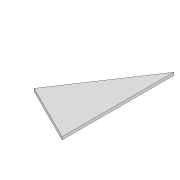
# Autodesk Inventor part: marker
Saved by Autodesk Inventor 2022 (Build 260153000, 153)
## iProperties
Created: 2022-09-01
Part Number: marker
Material: Generic
Document SubType Name: Modeling
Designer: Daniel
Density: 1 g/cm^3
Appearance: Default
Author: Daniel
Autodesk Inventor part; units mm, degrees
ref_plane "YZ Plane" through (0, 0, 0) normal (1, 0, 0) x (0, 1, 0)
ref_plane "XZ Plane" through (0, 0, 0) normal (0, 1, 0) x (-1, 0, 0)
ref_plane "XY Plane" through (0, 0, 0) normal (0, 0, 1) x (1, 0, 0)
sketch "Sketch1" plane through (0, 0, 0) normal (0, 1, 0) x (-1, 0, 0)
  line L0 (0, 0) -> (0, -2)
  line L1 (0, -2) -> (1, -0.5)
  line L2 (1, -0.5) -> (0, 0)
  dimension "d0" = 2
  dimension "d1" = 1
  dimension "d2" = 1.5
  constraints: 6 end point, 1 vertical
  measures "d0" distance of L0.start L0.end
  measures "d1" horizontal distance of L1.end L0.start
  measures "d2" vertical distance of L0.end L1.end
extrude "Extrusion1" add sketch "Sketch1" along normal blind 0.05
body "Solid1"
